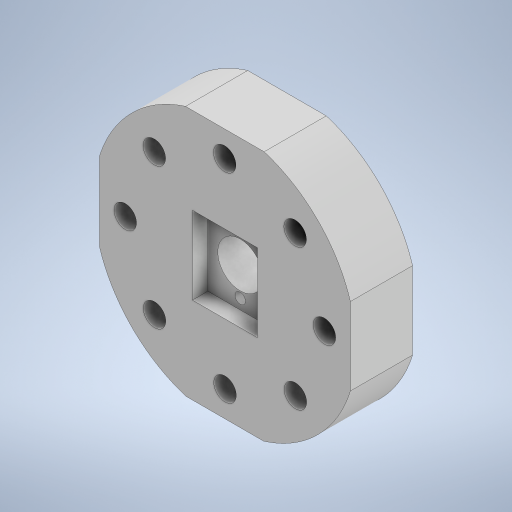
# Autodesk Inventor part: GripperBaseCircularUpper
Saved by Autodesk Inventor 2023 (Build 270158000, 158)
## iProperties
Created: 2023-06-03
Part Number: GripperBaseCircularUpper
Material: Ogólny
Document SubType Name: Modeling
Designer: Kamil
Density: 1 g/cm^3
Appearance: Domyślna
Author: Kamil
Autodesk Inventor part; units mm, degrees
ref_plane "YZ Plane" through (0, 0, 0) normal (1, 0, 0) x (0, 1, 0)
ref_plane "XZ Plane" through (0, 0, 0) normal (0, 1, 0) x (-1, 0, 0)
ref_plane "XY Plane" through (0, 0, 0) normal (0, 0, 1) x (1, 0, 0)
sketch "Szkic1" plane through (0, 0, 0) normal (0, 0, 1) x (1, 0, 0)
  line L0 (24.72, -24.72) -> (24.72, -14.42)
  line L1 (25.2197, -24.72) -> (24.72, -24.72)
  line L2 (24.72, -14.42) -> (25.2197, -14.42)
  line L3 (0, -39.14) -> (10.3, -39.14)
  line L4 (-14.42, -14.42) -> (-14.42, -24.72)
  line L5 (10.3, 0) -> (0, 0)
  line L6 (10.225, -25.645) -> (10.225, -13.495)
  line L7 (10.225, -25.645) -> (0.075, -25.645)
  line L8 (0.075, -13.495) -> (0.075, -25.645)
  line L9 (0.075, -13.495) -> (10.225, -13.495)
  line L10 (-14.9619, -24.72) -> (-14.9619, -24.7024)
  arc A0 (-14.9619, -24.7024) -> (0.075, -39.676) centre (5.1314, -19.5612) ccw
  arc A1 (10.3, -39.6475) -> (25.2201, -24.72) centre (5.1314, -19.5612) ccw
  line L11 (-14.9619, -14.42) -> (-14.42, -14.42)
  line L12 (24.72, -14.42) -> (25.2247, -14.42)
  line L13 (-14.42, -24.72) -> (-14.9619, -24.72)
  line L14 (0.075, -39.14) -> (0.075, -39.676)
  line L15 (0.075, 0.5536) -> (0.075, 0)
  line L16 (0.075, -13.495) -> (0.075, -25.645)
  line L17 (10.3, -39.6475) -> (10.3, -39.14)
  line L18 (10.3, 0) -> (10.3, 0.5251)
  line L19 (25.2201, -24.72) -> (24.72, -24.72)
  arc A2 (25.2247, -14.42) -> (10.3, 0.5251) centre (5.1314, -19.5612) ccw
  arc A3 (0.075, 0.5536) -> (-14.9619, -14.42) centre (5.1314, -19.5612) ccw
  circle A4 centre (5.1581, -35.1055) radius 1.75
  circle A5 centre (16.1418, -30.5337) radius 1.75
  circle A6 centre (20.6757, -19.5344) radius 1.75
  circle A7 centre (16.1039, -8.5508) radius 1.75
  circle A8 centre (5.1046, -4.0169) radius 1.75
  circle A9 centre (-5.879, -8.5887) radius 1.75
  circle A10 centre (-10.4129, -19.588) radius 1.75
  circle A11 centre (-5.8412, -30.5716) radius 1.75
  point P0 (5.15, -19.57)
  point P1 (-14.9574, -24.72)
  dimension "d0" = 3.5
  dimension "d3" = 360
  constraints: 40 end point, 12 centre point, 10 parallel, 8 point on circle, 2 horizontal, 2 point on line, 1 coincident, 17 other
  measures "d0" diameter of A4
extrude "Wyciągnięcie proste1" add sketch "Szkic1" along normal blind 9.7 contours L1 A1 L17 L3 L14 A0 L13 L4 L11 A3 L15 L5 L18 A2 L12 L2 L0
sketch "Szkic2" plane through (0, 0, 0) normal (0, 0, -1) x (-1, 0, 0)
  circle A0 centre (-16.1039, -8.5508) radius 1.75 projected
  circle A1 centre (-16.1039, -8.5508) radius 3
  arc A2 (-10.3, 0.5251) -> (-25.2247, -14.42) centre (-5.1314, -19.5612) ccw projected
  arc A3 (-0.075, -39.676) -> (14.9574, -24.72) centre (-5.1314, -19.5612) ccw projected
  circle A4 centre (-16.1418, -30.5337) radius 3
  circle A5 centre (5.8412, -30.5716) radius 3
  circle A6 centre (5.879, -8.5887) radius 3
  point P0 (0, 0)
  dimension "d7" = 6
  dimension "d10" = 360
  constraints: 4 centre point, 1 coincident, 9 other
  measures "d7" diameter of A1
extrude "Wyciągnięcie proste2" cut sketch "Szkic2" against normal blind 3.7
sketch "Szkic3" plane through (0, 0, 0) normal (0, 0, -1) x (-1, 0, 0)
  circle A0 centre (5.8412, -30.5716) radius 3 projected
  circle A1 centre (5.879, -8.5887) radius 3 projected
  circle A2 centre (-16.1418, -30.5337) radius 3 projected
  circle A3 centre (-16.1039, -8.5508) radius 3 projected
  line L0 (-24.72, -14.42) -> (-25.2247, -14.42) projected
  line L1 (-24.72, -24.72) -> (-24.72, -14.42) projected
  line L2 (-25.2201, -24.72) -> (-24.72, -24.72) projected
  arc A4 (-25.2201, -24.72) -> (-10.3, -39.6475) centre (-5.1314, -19.5612) ccw projected
  line L3 (-10.3, -39.14) -> (-10.3, -39.6475) projected
  line L4 (-0.075, -39.14) -> (-10.3, -39.14) projected
  line L5 (-0.075, -39.676) -> (-0.075, -39.14) projected
  arc A5 (-0.075, -39.676) -> (14.9574, -24.72) centre (-5.1314, -19.5612) ccw projected
  line L6 (14.42, -24.72) -> (14.9574, -24.72) projected
  line L7 (14.42, -14.42) -> (14.42, -24.72) projected
  line L8 (14.9619, -14.42) -> (14.42, -14.42) projected
  arc A6 (14.9619, -14.42) -> (-0.075, 0.5536) centre (-5.1314, -19.5612) ccw projected
  line L9 (-0.075, 0) -> (-0.075, 0.5536) projected
  line L10 (-10.3, 0) -> (-0.075, 0) projected
  line L11 (-10.3, 0.5251) -> (-10.3, 0) projected
  arc A7 (-10.3, 0.5251) -> (-25.2247, -14.42) centre (-5.1314, -19.5612) ccw projected
  circle A8 centre (10.4129, -19.588) radius 1.75 projected
  circle A9 centre (-5.1581, -35.1055) radius 1.75 projected
  circle A10 centre (-20.6757, -19.5344) radius 1.75 projected
  circle A11 centre (-5.1046, -4.0169) radius 1.75 projected
  line L12 (-10.225, -25.645) -> (-0.075, -25.645) projected
  line L13 (-10.225, -13.495) -> (-10.225, -25.645) projected
  line L14 (-0.075, -13.495) -> (-10.225, -13.495) projected
  line L15 (-0.075, -25.645) -> (-0.075, -13.495) projected
  line L16 (-10.225, -13.495) -> (-8.225, -13.495)
  line L17 (-8.225, -13.495) -> (-8.225, -25.645)
  line L18 (-8.225, -25.645) -> (-10.225, -25.645)
  line L19 (-10.225, -25.645) -> (-10.225, -13.495)
  line L20 (-0.075, -25.645) -> (-2.075, -25.645)
  line L21 (-2.075, -25.645) -> (-2.075, -13.495)
  line L22 (-2.075, -13.495) -> (-0.075, -13.495)
  line L23 (-0.075, -13.495) -> (-0.075, -25.645)
  point P0 (0, 0)
  dimension "d14" = 2
  dimension "d15" = 2
  constraints: 16 end point, 4 parallel, 2 horizontal, 2 perpendicular, 2 point on line
  measures "d14" distance of L17.end L18.end
  measures "d15" distance of L21.end L22.end
extrude "Wyciągnięcie proste3" add sketch "Szkic3" against normal blind 4.7 contours L13 L14 L17 L12 | L21 L14 L15 L12
sketch "Szkic4" plane through (0, 0, 9.7) normal (0, 0, 1) x (1, 0, 0)
  line L0 (24.72, -14.42) -> (25.2247, -14.42) projected
  arc A0 (25.2247, -14.42) -> (10.3, 0.5251) centre (5.1314, -19.5612) ccw projected
  line L1 (10.3, 0.5251) -> (10.3, 0) projected
  line L2 (10.3, 0) -> (0.075, 0) projected
  line L3 (0.075, 0) -> (0.075, 0.5536) projected
  arc A1 (0.075, 0.5536) -> (-14.9619, -14.42) centre (5.1314, -19.5612) ccw projected
  line L4 (-14.9619, -14.42) -> (-14.42, -14.42) projected
  line L5 (-14.42, -14.42) -> (-14.42, -24.72) projected
  line L6 (-14.42, -24.72) -> (-14.9574, -24.72) projected
  arc A2 (-14.9574, -24.72) -> (0.075, -39.676) centre (5.1314, -19.5612) ccw projected
  line L7 (0.075, -39.676) -> (0.075, -39.14) projected
  line L8 (0.075, -39.14) -> (10.3, -39.14) projected
  line L9 (10.3, -39.14) -> (10.3, -39.6475) projected
  arc A3 (10.3, -39.6475) -> (25.2201, -24.72) centre (5.1314, -19.5612) ccw projected
  line L10 (25.2201, -24.72) -> (24.72, -24.72) projected
  line L11 (24.72, -24.72) -> (24.72, -14.42) projected
  circle A4 centre (-10.4129, -19.588) radius 1.75 projected
  circle A5 centre (5.1581, -35.1055) radius 1.75 projected
  circle A6 centre (20.6757, -19.5344) radius 1.75 projected
  circle A7 centre (5.1046, -4.0169) radius 1.75 projected
  circle A8 centre (-5.8412, -30.5716) radius 1.75 projected
  circle A9 centre (-5.879, -8.5887) radius 1.75 projected
  circle A10 centre (16.1039, -8.5508) radius 1.75 projected
  circle A11 centre (16.1418, -30.5337) radius 1.75 projected
  line L12 (10.225, -25.645) -> (0.075, -25.645) projected
  line L13 (0.075, -25.645) -> (0.075, -13.495) projected
  line L14 (0.075, -13.495) -> (10.225, -13.495) projected
  line L15 (10.225, -13.495) -> (10.225, -25.645) projected
  line L16 (10.3, 0.5251) -> (10.3, 0) projected
  line L17 (10.3, 0.5251) -> (0.075, 0.5536)
  line L18 (10.3, 0) -> (0.075, 0) projected
  circle A12 centre (5.1314, -19.5612) radius 20.2325
  point P0 (0, 0)
  point P1 (-14.4371, -14.42)
  point P2 (0.075, 0.0293)
  point P3 (0.075, -39.1517)
  point P4 (-14.4324, -24.72)
  point P5 (24.72, -24.6249)
  point P6 (10.2329, -39.14)
  point P7 (24.72, -14.4975)
  constraints: 2 end point, 1 coincident, 3 other
extrude "Wyciągnięcie proste4" cut sketch "Szkic4" against normal through all contours L11 A12 L1 A0 L0 | L11 L10 A3 L9 L8 A12 | L7 A2 L6 A12 | A12 L4 A1 L3
sketch "Szkic5" plane through (0, 0, 0) normal (0, 0, -1) x (-1, 0, 0)
  line L0 (-10.225, -13.495) -> (-10.225, -25.645) projected
  line L1 (-8.225, -13.495) -> (-10.225, -13.495) projected
  line L2 (-2.075, -13.495) -> (-8.225, -13.495) projected
  line L3 (-0.075, -13.495) -> (-2.075, -13.495) projected
  line L4 (-0.075, -25.645) -> (-0.075, -13.495) projected
  line L5 (-2.075, -25.645) -> (-0.075, -25.645) projected
  line L6 (-8.225, -25.645) -> (-2.075, -25.645) projected
  line L7 (-10.225, -25.645) -> (-8.225, -25.645) projected
  line L8 (-10.2317, -25.6607) -> (-10.2317, -13.4607)
  line L9 (-0.0317, -13.4607) -> (-10.2317, -13.4607)
  circle A0 centre (-5.1314, -15.0608) radius 0.8097
  line L10 (-0.0317, -25.6607) -> (-0.0317, -13.4607)
  line L11 (-10.2317, -25.6607) -> (-0.0317, -25.6607)
  circle A1 centre (-5.1314, -19.5612) radius 3.4994
  circle A2 centre (-5.1314, -24.061) radius 0.8096
  arc A3 (-10.3, 0) -> (-24.72, -14.4975) centre (-5.1314, -19.5612) ccw projected
  point P0 (0, 0)
  point P1 (-5.1317, -19.5607)
  constraints: 8 end point, 3 centre point
extrude "Wyciągnięcie proste5" cut sketch "Szkic5" against normal through all contours L1 L2 L3 L4 L5 L6 L7 L0 | A1
extrude "Wyciągnięcie proste6" add sketch "Szkic5" against normal blind 7.3 contours L1 L2 L3 L4 L5 L6 L7 L0
sketch "Szkic6" plane through (0, 0, 0) normal (0, 0, -1) x (-1, 0, 0)
  arc A0 (-10.3, 0) -> (-24.72, -14.4975) centre (-5.1314, -19.5612) ccw projected
  circle A1 centre (-5.1314, -19.5612) radius 3.4994 projected
  circle A2 centre (-5.1314, -19.5612) radius 20.5
  circle A3 centre (-5.1314, -24.061) radius 0.8096 projected
  circle A4 centre (-5.1314, -19.5612) radius 3.4994 projected
  circle A5 centre (-5.1314, -15.0608) radius 0.8097 projected
  circle A6 centre (-5.1046, -4.0169) radius 1.75 projected
  circle A7 centre (-20.6757, -19.5344) radius 1.75 projected
  circle A8 centre (-5.1581, -35.1055) radius 1.75 projected
  circle A9 centre (10.4129, -19.588) radius 1.75 projected
  circle A10 centre (-16.1039, -8.5508) radius 3 projected
  circle A11 centre (-16.1418, -30.5337) radius 3 projected
  circle A12 centre (5.879, -8.5887) radius 3 projected
  circle A13 centre (5.8412, -30.5716) radius 3 projected
  arc A14 (-0.075, -39.1517) -> (14.4324, -24.72) centre (-5.1314, -19.5612) ccw projected
  line L0 (14.42, -24.72) -> (14.4324, -24.72) projected
  line L1 (14.42, -14.42) -> (14.42, -24.72) projected
  line L2 (14.4371, -14.42) -> (14.42, -14.42) projected
  arc A15 (14.4371, -14.42) -> (-0.075, 0.0293) centre (-5.1314, -19.5612) ccw projected
  line L3 (-0.075, 0) -> (-0.075, 0.0293) projected
  line L4 (-10.3, 0) -> (-0.075, 0) projected
  arc A16 (-10.3, 0) -> (-24.72, -14.4975) centre (-5.1314, -19.5612) ccw projected
  line L5 (-24.72, -24.6249) -> (-24.72, -14.4975) projected
  arc A17 (-24.72, -24.6249) -> (-10.2329, -39.14) centre (-5.1314, -19.5612) ccw projected
  line L6 (-0.075, -39.14) -> (-10.2329, -39.14) projected
  line L7 (-0.075, -39.1517) -> (-0.075, -39.14) projected
  line L8 (-24.72, -6.5254) -> (-24.72, -33.3555)
  line L9 (14.4371, -5.2931) -> (14.4371, -36.8555)
  line L10 (-20.6757, -39.1517) -> (13.3882, -39.1517)
  line L11 (-24, 0) -> (14, 0)
  point P0 (0, 0)
  point P1 (-24.72, -25.6056)
  point P2 (-11.1697, -39.1517)
  point P3 (-0.075, -39.1517)
  point P4 (-0.075, -39.1517)
  point P5 (0.907, -39.1517)
  point P6 (14.4371, -25.6707)
  point P7 (1.0013, 0)
  point P8 (0.0373, 0)
  point P9 (14.4371, -13.4517)
  point P10 (-11.264, 0)
  point P11 (-24.72, -13.5168)
  dimension "d24" = 41
  constraints: 8 end point, 2 horizontal, 2 vertical, 1 centre point, 1 coincident
  measures "d24" diameter of A2
extrude "Wyciągnięcie proste7" add sketch "Szkic6" against normal up to surface (9.7 mm away) contours A0 L8 A2 L11 | A17 L6 L7 L10 A2 L8 | L11 A2 L9 A15 | L9 A2 L10 A14 L0 L1 L2
sketch "Szkic7" plane through (0, 0, 9.7) normal (0, 0, 1) x (1, 0, 0)
  line L0 (10.225, -25.645) -> (0.075, -25.645) projected
  line L1 (0.075, -25.645) -> (0.075, -13.495) projected
  line L2 (0.075, -13.495) -> (10.225, -13.495) projected
  line L3 (10.225, -13.495) -> (10.225, -25.645) projected
  circle A0 centre (16.1418, -30.5337) radius 1.75 projected
  circle A1 centre (16.1039, -8.5508) radius 1.75 projected
  circle A2 centre (-5.879, -8.5887) radius 1.75 projected
  circle A3 centre (-5.8412, -30.5716) radius 1.75 projected
  circle A4 centre (5.1046, -4.0169) radius 1.75 projected
  circle A5 centre (20.6757, -19.5344) radius 1.75 projected
  circle A6 centre (5.1581, -35.1055) radius 1.75 projected
  circle A7 centre (-10.4129, -19.588) radius 1.75 projected
  line L4 (24.72, -13.5168) -> (24.72, -25.6056) projected
  arc A8 (24.72, -13.5168) -> (11.264, 0) centre (5.1314, -19.5612) ccw projected
  line L5 (0.075, 0) -> (11.264, 0) projected
  line L6 (0.075, 0) -> (0.075, 0.0293) projected
  arc A9 (0.075, 0.0293) -> (-0.0373, 0) centre (5.1314, -19.5612) ccw projected
  line L7 (-1.0013, 0) -> (-0.0373, 0) projected
  arc A10 (-1.0013, 0) -> (-14.4371, -13.4517) centre (5.1314, -19.5612) ccw projected
  line L8 (-14.4371, -25.6707) -> (-14.4371, -13.4517) projected
  arc A11 (-14.4371, -25.6707) -> (-0.907, -39.1517) centre (5.1314, -19.5612) ccw projected
  line L9 (11.1697, -39.1517) -> (-0.907, -39.1517) projected
  arc A12 (11.1697, -39.1517) -> (24.72, -25.6056) centre (5.1314, -19.5612) ccw projected
  line L10 (0.075, 0) -> (-0.0373, 0)
  point P0 (0, 0)
  constraints: 2 end point, 1 horizontal
extrude "Wyciągnięcie proste8" cut sketch "Szkic7" against normal through all contours L10 A9 L6
